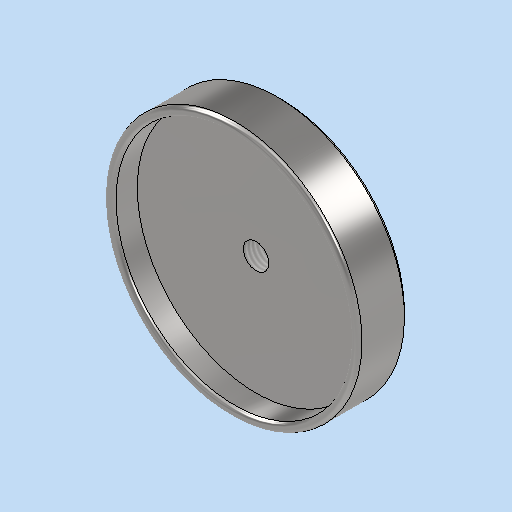
# Autodesk Inventor part: boron-bowl
Saved by Autodesk Inventor 2025 (Build 290162000, 162)
## iProperties
Created: 2024-07-17
Part Number: boron-bowl
Material: Stainless Steel
Document SubType Name: Modeling
Designer: kuzmin
Density: 8 g/cm^3
Appearance: Semi-Polished
Author: kuzmin
Autodesk Inventor part; units mm, degrees
ref_plane "YZ Plane" through (0, 0, 0) normal (1, 0, 0) x (0, 1, 0)
ref_plane "XZ Plane" through (0, 0, 0) normal (0, 1, 0) x (-1, 0, 0)
ref_plane "XY Plane" through (0, 0, 0) normal (0, 0, 1) x (1, 0, 0)
sketch "Sketch1" plane through (0, 0, 0) normal (1, 0, 0) x (0, 1, 0)
  line L0 (0, 0) -> (0, 6)
  line L1 (0, 6) -> (14, 6) construction
  line L2 (14, 6) -> (15, 6)
  line L3 (15, 6) -> (15, 0)
  line L4 (15, 0) -> (0, 0)
  line L5 (14, 6) -> (14, 3)
  line L6 (14, 3) -> (0, 3)
  dimension "d0" = 30
  dimension "d1" = 6
  dimension "d2" = 3
  dimension "d3" = 1
  constraints: 14 end point, 4 perpendicular, 2 vertical, 1 midpoint, 1 point on line
  measures "d0" diameter of L3 L0
  measures "d1" distance of L2.end L3.end
  measures "d2" distance between parallel lines of L4 L6
  measures "d3" distance of L1.end L2.end
revolve "Revolution1" add sketch "Sketch1" angle 360 about axis through (0, 0, 0) along (0, 0, 1)
chamfer "Chamfer1" distance 0.5 angle 45 1 edges at (0, -15, 0)
sketch "Sketch2" plane through (0, 0, 0) normal (0, 0, -1) x (-1, 0, 0)
  point P0 (0, 0)
  point P1 (0, 0)
  constraints: 1 coincident
hole "Hole1" at (0, 0, 0) direction (0, 0, 1) diameter 3 end through all
thread "Thread1" size "M3x0.5" class "6H" standard "ANSI Metric M Profile" full length
fillet "Fillet1" radius 0.5 2 edges at (0, -15, 6) (0, -14, 6)
body "Solid1"
